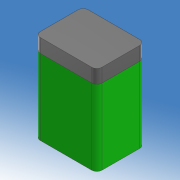
# Autodesk Inventor part: Li-Iron-Phosphate Battery
Saved by Autodesk Inventor 2020 (Build 240168000, 168)
## iProperties
Created: 2019-10-09
Part Number: Li-Iron-Phosphate Battery
Material: Generic
Document SubType Name: Modeling
Designer: mpark
Density: 1 g/cm^3
Appearance: Default
Author: mpark
Autodesk Inventor part; units mm, degrees
ref_plane "YZ Plane" through (0, 0, 0) normal (1, 0, 0) x (0, 1, 0)
ref_plane "XZ Plane" through (0, 0, 0) normal (0, 1, 0) x (-1, 0, 0)
sketch "Sketch1" plane through (0, 0, 0) normal (1, 0, 0) x (0, 1, 0)
  line L0 (165.1, 44.45) -> (0, 44.45)
  line L1 (0, 44.45) -> (0, -44.45)
  line L2 (0, -44.45) -> (165.1, -44.45)
  line L3 (165.1, -44.45) -> (165.1, 44.45)
  point P0 (0, 0)
  point P1 (165.1, 0)
  point P2 (0, 0)
  dimension "d0" = 88.9
  dimension "d1" = 165.1
  constraints: 8 end point, 2 midpoint, 2 parallel, 1 coincident, 1 horizontal, 1 horizontal alignment, 1 perpendicular
  measures "d0" distance of L2.end L0.start
  measures "d1" distance between parallel lines of L1 L3
extrude "Extrusion1" add sketch "Sketch1" along normal mid plane 114.3
ref_plane "Work Plane1" through (-57.15, 139.7, 44.45) normal (0, 1, 0) x (1, 0, 0)
split body "Split1" result two bodies by plane through (-57.15, 139.7, 44.45) normal (0, 1, 0) first body at (-19.05, 164.6, -14.8167)
fillet "Fillet1" radius 9.525 8 edges at (-57.15, 152.4, 44.45) (57.15, 152.4, 44.45) (57.15, 152.4, -44.45) (-57.15, 152.4, -44.45) (-57.15, 69.85, 44.45) (57.15, 69.85, 44.45) (57.15, 69.85, -44.45) (-57.15, 69.85, -44.45)
body "Solid2"
body "Solid3"
